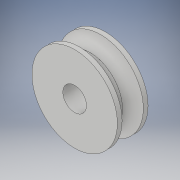
# Autodesk Inventor part: pulley alpha
Saved by Autodesk Inventor 2019 (Build 230136000, 136)
## iProperties
Created: 2018-11-14
Part Number: pulley alpha
Material: Generic
Document SubType Name: Modeling
Designer: Delta
Density: 1 g/cm^3
Appearance: Default
Author: Delta
Autodesk Inventor part; units mm, degrees
ref_plane "YZ Plane" through (0, 0, 0) normal (1, 0, 0) x (0, 1, 0)
ref_plane "XZ Plane" through (0, 0, 0) normal (0, 1, 0) x (-1, 0, 0)
ref_plane "XY Plane" through (0, 0, 0) normal (0, 0, 1) x (1, 0, 0)
sketch "Sketch1" plane through (0, 0, 0) normal (0, 0, 1) x (1, 0, 0)
  circle A0 centre (0, 0) radius 9.1821
  dimension "d0" = 18.3642
  constraints: 1 centre point, 1 coincident
  measures "d0" diameter of A0
extrude "Extrusion1" add sketch "Sketch1" along normal blind 1.016
sketch "Sketch2" plane through (0, 0, 1.016) normal (0, 0, 1) x (1, 0, 0)
  circle A0 centre (0, 0) radius 6.985
  dimension "d3" = 13.97
  constraints: 1 centre point, 1 coincident
  measures "d3" diameter of A0
extrude "Extrusion2" add sketch "Sketch2" along normal blind 2.286
sketch "Sketch3" plane through (0, 0, 3.302) normal (0, 0, 1) x (1, 0, 0)
  point P0 (0, 0)
hole "Hole1" at (0, 0, 3.302) direction (0, 0, -1) diameter 5.08 depth 25.4 tip angle 118
mirror "Mirror1" about plane through (0, 0, 3.302) normal (0, 0, 1) of "Extrusion2", "Extrusion1", "Hole1"
fillet "Fillet1" radius 2.286 2 edges at (-6.985, 0, 1.016) (-6.985, 0, 5.588)
body "Solid1"
